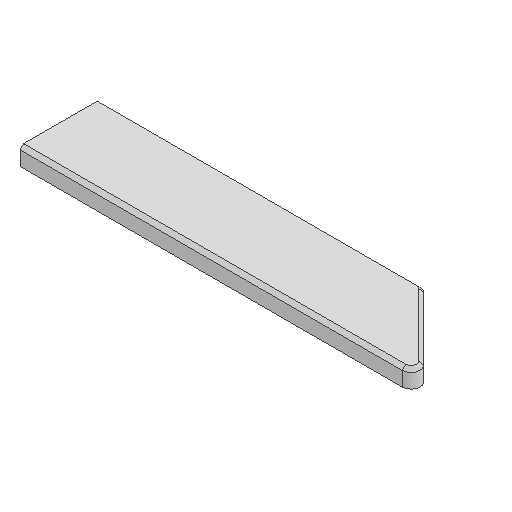
# Autodesk Inventor part: Border
Saved by Autodesk Inventor 2025.2 (Build 292293000, 293)
## iProperties
Created: 2025-03-03
Part Number: Border
Material: Generic
Document SubType Name: Modeling
Designer: Marcu
Density: 1 g/cm^3
Appearance: Default
Author: Marcu
Autodesk Inventor part; units mm, degrees
ref_plane "YZ Plane" through (0, 0, 0) normal (1, 0, 0) x (0, 1, 0)
ref_plane "XZ Plane" through (0, 0, 0) normal (0, 1, 0) x (-1, 0, 0)
ref_plane "XY Plane" through (0, 0, 0) normal (0, 0, 1) x (1, 0, 0)
sketch "Sketch1" plane through (0, 0, 0) normal (0, 0, 1) x (1, 0, 0)
  line L0 (-180, 0) -> (0, 0)
  line L1 (-225, -45) -> (0, -45)
  line L2 (-180, 0) -> (-225, -45)
  line L3 (0, 0) -> (0, -45)
  dimension "d2" = 45
  dimension "d9" = 225
  dimension "d10" = 180
  constraints: 8 end point, 1 horizontal, 1 parallel
  measures "d2" distance between parallel lines of L0 L1
  measures "d9" distance of L1.start L1.end
  measures "d10" distance of L0.start point (0, 0)
extrude "Extrusion1" add sketch "Sketch1" along normal blind 10
sketch "Sketch4" plane through (0, 0, 0) normal (0, 0, -1) x (-1, 0, 0)
  circle A0 centre (22.5, -22.5) radius 7.5
  circle A1 centre (157.5, -22.5) radius 7.5
  point P0 (0, -45)
  point P1 (180, 0)
  dimension "d26" = 15
  dimension "d30" = 15
  constraints: 2 centre point
  measures "d26" diameter of A0
  measures "d30" diameter of A1
extrude "Extrusion2" add sketch "Sketch4" along normal blind 10
fillet "Fillet5" radius 5 2 edges at (-225, -45, 5) (-180, 0, 5)
chamfer "Chamfer3" distance 2 angle 45 5 edges at (-106.4645, -45, 10) (-217.5483, -41.9134, 10) (-198.9645, -18.9645, 10) (-179.8423, -0.3806, 10) (-88.9645, 0, 10)
mirror "Mirror1" about plane through (0, 0, 0) normal (1, 0, 0)
sketch "Sketch6" plane through (0, 0, 10) normal (0, 0, 1) x (1, 0, 0)
  line L0 (0, 20) -> (-220, 20)
  line L1 (-220, 20) -> (-220, -60)
  line L2 (-220, -60) -> (0, -60)
  line L3 (0, -60) -> (0, 20)
  point P0 (0, 0)
  dimension "d47" = 220
  dimension "d48" = 80
  constraints: 8 end point, 2 parallel, 1 horizontal, 1 perpendicular
  measures "d47" distance of L2.end L1.end
  measures "d48" distance of L1.end L0.end
extrude "Extrusion6" cut sketch "Sketch6" against normal blind 20
body "Solid1"
